Autodesk Inventor part; units mm, degrees
(part 2 of 2)
  arc A534 (36.3761, 13.3545) -> (36.8733, 13.0276) centre (36.8454, 13.5269) ccw
  arc A535 (36.3761, 13.3545) -> (36.3337, 13.4695) centre (0, 0) ccw
  arc A536 (36.4994, 14.041) -> (36.3337, 13.4695) centre (36.8025, 13.6433) ccw
  arc A537 (37.1579, 14.5094) -> (36.4994, 14.041) centre (43.9592, 4.2516) ccw
  arc A538 (37.1579, 14.5094) -> (37.2486, 14.5788) centre (36.7, 15.2016) ccw
  arc A539 (37.2486, 14.5788) -> (37.9831, 15.2771) centre (28.4355, 24.5841) ccw
  arc A540 (37.9831, 15.2771) -> (38.0042, 15.3845) centre (37.9115, 15.3469) ccw
  arc A541 (38.0042, 15.3845) -> (37.7515, 15.9946) centre (0, 0) ccw
  arc A542 (37.7515, 15.9946) -> (37.6607, 16.0555) centre (37.6594, 15.9556) ccw
  arc A543 (37.6607, 16.0555) -> (36.6475, 16.03) centre (37.4905, 2.7233) ccw
  arc A544 (36.6475, 16.03) -> (36.5343, 16.0149) centre (36.7, 15.2016) ccw
  arc A545 (35.7375, 15.8805) -> (36.5343, 16.0149) centre (34.0902, 28.0775) ccw
  arc A546 (35.2162, 16.1674) -> (35.7375, 15.8805) centre (35.6706, 16.376) ccw
  arc A547 (35.2162, 16.1674) -> (35.1649, 16.2787) centre (0, 0) ccw
  arc A548 (35.2853, 16.8614) -> (35.1649, 16.2787) centre (35.6186, 16.4887) ccw
  arc A549 (35.905, 17.38) -> (35.2853, 16.8614) centre (43.4901, 7.6875) ccw
  arc A550 (35.905, 17.38) -> (35.9899, 17.4564) centre (35.3942, 18.0342) ccw
  arc A551 (35.9899, 17.4564) -> (36.6674, 18.2102) centre (26.419, 26.7394) ccw
  arc A552 (36.6674, 18.2102) -> (36.68, 18.3188) centre (36.5905, 18.2741) ccw
  arc A553 (36.68, 18.3188) -> (36.3802, 18.9072) centre (0, 0) ccw
  arc A554 (36.3802, 18.9072) -> (36.2849, 18.9609) centre (36.2914, 18.8611) ccw
  arc A555 (36.2849, 18.9609) -> (35.2769, 18.8559) centre (37.1613, 5.6564) ccw
  arc A556 (35.2769, 18.8559) -> (35.1652, 18.832) centre (35.3942, 18.0342) ccw
  arc A557 (34.3813, 18.6355) -> (35.1652, 18.832) centre (31.7822, 30.6656) ccw
  arc A558 (33.8391, 18.8806) -> (34.3813, 18.6355) centre (34.2757, 19.1242) ccw
  arc A559 (33.8391, 18.8806) -> (33.7792, 18.9875) centre (0, 0) ccw
  arc A560 (33.8536, 19.5779) -> (33.7792, 18.9875) centre (34.2151, 19.2325) ccw
  arc A561 (34.4306, 20.1435) -> (33.8536, 19.5779) centre (42.7529, 11.076) ccw
  arc A562 (34.4306, 20.1435) -> (34.5094, 20.2263) centre (33.8701, 20.7556) ccw
  arc A563 (34.5094, 20.2263) -> (35.1256, 21.0309) centre (24.2396, 28.7298) ccw
  arc A564 (35.1256, 21.0309) -> (35.1296, 21.1402) centre (35.044, 21.0887) ccw
  arc A565 (35.1296, 21.1402) -> (34.7846, 21.7033) centre (0, 0) ccw
  arc A566 (34.7846, 21.7033) -> (34.6854, 21.7493) centre (34.6998, 21.6503) ccw
  arc A567 (34.6854, 21.7493) -> (33.6887, 21.5655) centre (36.6029, 8.5546) ccw
  arc A568 (33.6887, 21.5655) -> (33.5792, 21.533) centre (33.8701, 20.7556) ccw
  arc A569 (32.8132, 21.2756) -> (33.5792, 21.533) centre (29.2782, 33.0647) ccw
  arc A570 (32.2534, 21.4774) -> (32.8132, 21.2756) centre (32.6696, 21.7545) ccw
  arc A571 (32.2534, 21.4774) -> (32.1854, 21.5793) centre (0, 0) ccw
  arc A572 (32.2131, 22.1737) -> (32.1854, 21.5793) centre (32.6007, 21.8577) ccw
  arc A573 (32.7441, 22.7828) -> (32.2131, 22.1737) centre (41.7521, 14.3962) ccw
  arc A574 (32.7441, 22.7828) -> (32.8161, 22.8715) centre (32.1372, 23.3491) ccw
  arc A575 (32.8161, 22.8715) -> (33.3673, 23.722) centre (21.9107, 30.543) ccw
  arc A576 (33.3673, 23.722) -> (33.3627, 23.8313) centre (33.2813, 23.7732) ccw
  arc A577 (33.3627, 23.8313) -> (32.9745, 24.3655) centre (0, 0) ccw
  arc A578 (32.9745, 24.3655) -> (32.872, 24.4036) centre (32.8941, 24.3061) ccw
  arc A579 (32.872, 24.4036) -> (31.8928, 24.1422) centre (35.8189, 11.4) ccw
  arc A580 (31.8928, 24.1422) -> (31.7862, 24.1012) centre (32.1372, 23.3491) ccw
  arc A581 (31.0428, 23.7845) -> (31.7862, 24.1012) centre (26.5937, 35.2599) ccw
  arc A582 (30.4689, 23.9418) -> (31.0428, 23.7845) centre (30.8621, 24.2507) ccw
  arc A583 (30.4689, 23.9418) -> (30.3931, 24.038) centre (0, 0) ccw
  arc A584 (30.3741, 24.6327) -> (30.3931, 24.038) centre (30.7852, 24.3481) ccw
  arc A585 (30.8556, 25.2817) -> (30.3741, 24.6327) centre (40.4939, 17.6277) ccw
  arc A586 (30.8556, 25.2817) -> (30.9204, 25.3757) centre (30.2062, 25.7985) ccw
  arc A587 (30.9204, 25.3757) -> (31.4032, 26.2668) centre (19.4468, 32.168) ccw
  arc A588 (31.4032, 26.2668) -> (31.3901, 26.3754) centre (31.3135, 26.3111) ccw
  arc A589 (31.3901, 26.3754) -> (30.9612, 26.8776) centre (0, 0) ccw
  arc A590 (30.9612, 26.8776) -> (30.856, 26.9075) centre (30.8857, 26.812) ccw
  arc A591 (30.856, 26.9075) -> (29.9003, 26.5701) centre (34.8141, 14.1752) ccw
  arc A592 (29.9003, 26.5701) -> (29.7973, 26.5208) centre (30.2062, 25.7985) ccw
  arc A593 (29.081, 26.1468) -> (29.7973, 26.5208) centre (23.7453, 37.2377) ccw
  arc A594 (28.4965, 26.2585) -> (29.081, 26.1468) centre (28.8642, 26.5973) ccw
  arc A595 (28.4965, 26.2585) -> (28.4134, 26.3485) centre (0, 0) ccw
  arc A596 (28.3478, 26.9399) -> (28.4134, 26.3485) centre (28.78, 26.6885) ccw
  arc A597 (28.7769, 27.6246) -> (28.3478, 26.9399) centre (38.986, 20.7505) ccw
  arc A598 (28.7769, 27.6246) -> (28.8341, 27.7235) centre (28.089, 28.089) ccw
  arc A599 (28.8341, 27.7235) -> (29.2455, 28.6497) centre (16.863, 33.5946) ccw
  arc A600 (29.2455, 28.6497) -> (29.2239, 28.757) centre (29.1526, 28.6868) ccw
  arc A601 (29.2239, 28.757) -> (28.757, 29.2239) centre (0, 0) ccw
  arc A602 (28.757, 29.2239) -> (28.6497, 29.2455) centre (28.6868, 29.1526) ccw
  arc A603 (28.6497, 29.2455) -> (27.7235, 28.8341) centre (33.5946, 16.863) ccw
  arc A604 (27.7235, 28.8341) -> (27.6246, 28.7769) centre (28.089, 28.089) ccw
  arc A605 (26.9399, 28.3478) -> (27.6246, 28.7769) centre (20.7505, 38.986) ccw
  arc A606 (26.3485, 28.4134) -> (26.9399, 28.3478) centre (26.6885, 28.78) ccw
  arc A607 (26.3485, 28.4134) -> (26.2585, 28.4965) centre (0, 0) ccw
  arc A608 (26.1468, 29.081) -> (26.2585, 28.4965) centre (26.5973, 28.8642) ccw
  arc A609 (26.5208, 29.7973) -> (26.1468, 29.081) centre (37.2377, 23.7453) ccw
  arc A610 (26.5208, 29.7973) -> (26.5701, 29.9003) centre (25.7985, 30.2062) ccw
  arc A611 (26.5701, 29.9003) -> (26.9075, 30.856) centre (14.1752, 34.8141) ccw
  arc A612 (26.9075, 30.856) -> (26.8776, 30.9612) centre (26.812, 30.8857) ccw
  arc A613 (26.8776, 30.9612) -> (26.3754, 31.3901) centre (0, 0) ccw
  arc A614 (26.3754, 31.3901) -> (26.2668, 31.4032) centre (26.3111, 31.3135) ccw
  arc A615 (26.2668, 31.4032) -> (25.3757, 30.9204) centre (32.168, 19.4468) ccw
  arc A616 (25.3757, 30.9204) -> (25.2817, 30.8556) centre (25.7985, 30.2062) ccw
  arc A617 (24.6327, 30.3741) -> (25.2817, 30.8556) centre (17.6277, 40.4939) ccw
  arc A618 (24.038, 30.3931) -> (24.6327, 30.3741) centre (24.3481, 30.7852) ccw
  arc A619 (24.038, 30.3931) -> (23.9418, 30.4689) centre (0, 0) ccw
  arc A620 (23.7845, 31.0428) -> (23.9418, 30.4689) centre (24.2507, 30.8621) ccw
  arc A621 (24.1012, 31.7862) -> (23.7845, 31.0428) centre (35.2599, 26.5937) ccw
  arc A622 (24.1012, 31.7862) -> (24.1422, 31.8928) centre (23.3491, 32.1372) ccw
  arc A623 (24.1422, 31.8928) -> (24.4036, 32.872) centre (11.4, 35.8189) ccw
  arc A624 (24.4036, 32.872) -> (24.3655, 32.9745) centre (24.3061, 32.8941) ccw
  arc A625 (24.3655, 32.9745) -> (23.8313, 33.3627) centre (0, 0) ccw
  arc A626 (23.8313, 33.3627) -> (23.722, 33.3673) centre (23.7732, 33.2813) ccw
  arc A627 (23.722, 33.3673) -> (22.8715, 32.8161) centre (30.543, 21.9107) ccw
  arc A628 (22.8715, 32.8161) -> (22.7828, 32.7441) centre (23.3491, 32.1372) ccw
  arc A629 (22.1737, 32.2131) -> (22.7828, 32.7441) centre (14.3962, 41.7521) ccw
  arc A630 (21.5793, 32.1854) -> (22.1737, 32.2131) centre (21.8577, 32.6007) ccw
  arc A631 (21.5793, 32.1854) -> (21.4774, 32.2534) centre (0, 0) ccw
  arc A632 (21.2756, 32.8132) -> (21.4774, 32.2534) centre (21.7545, 32.6696) ccw
  arc A633 (21.533, 33.5792) -> (21.2756, 32.8132) centre (33.0647, 29.2782) ccw
  arc A634 (21.533, 33.5792) -> (21.5655, 33.6887) centre (20.7556, 33.8701) ccw
  arc A635 (21.5655, 33.6887) -> (21.7493, 34.6854) centre (8.5546, 36.6029) ccw
  arc A636 (21.7493, 34.6854) -> (21.7033, 34.7846) centre (21.6503, 34.6998) ccw
  arc A637 (21.7033, 34.7846) -> (21.1402, 35.1296) centre (0, 0) ccw
  arc A638 (21.1402, 35.1296) -> (21.0309, 35.1256) centre (21.0887, 35.044) ccw
  arc A639 (21.0309, 35.1256) -> (20.2263, 34.5094) centre (28.7298, 24.2396) ccw
  arc A640 (20.2263, 34.5094) -> (20.1435, 34.4306) centre (20.7556, 33.8701) ccw
  arc A641 (19.5779, 33.8536) -> (20.1435, 34.4306) centre (11.076, 42.7529) ccw
  arc A642 (18.9875, 33.7792) -> (19.5779, 33.8536) centre (19.2325, 34.2151) ccw
  arc A643 (18.9875, 33.7792) -> (18.8806, 33.8391) centre (0, 0) ccw
  arc A644 (18.6355, 34.3813) -> (18.8806, 33.8391) centre (19.1242, 34.2757) ccw
  arc A645 (18.832, 35.1652) -> (18.6355, 34.3813) centre (30.6656, 31.7822) ccw
  arc A646 (18.832, 35.1652) -> (18.8559, 35.2769) centre (18.0342, 35.3942) ccw
  arc A647 (18.8559, 35.2769) -> (18.9609, 36.2849) centre (5.6564, 37.1613) ccw
  arc A648 (18.9609, 36.2849) -> (18.9072, 36.3802) centre (18.8611, 36.2914) ccw
  arc A649 (18.9072, 36.3802) -> (18.3188, 36.68) centre (0, 0) ccw
  arc A650 (18.3188, 36.68) -> (18.2102, 36.6674) centre (18.2741, 36.5905) ccw
  arc A651 (18.2102, 36.6674) -> (17.4564, 35.9899) centre (26.7394, 26.419) ccw
  arc A652 (17.4564, 35.9899) -> (17.38, 35.905) centre (18.0342, 35.3942) ccw
  arc A653 (16.8614, 35.2853) -> (17.38, 35.905) centre (7.6875, 43.4901) ccw
  arc A654 (16.2787, 35.1649) -> (16.8614, 35.2853) centre (16.4887, 35.6186) ccw
  arc A655 (16.2787, 35.1649) -> (16.1674, 35.2162) centre (0, 0) ccw
  arc A656 (15.8805, 35.7375) -> (16.1674, 35.2162) centre (16.376, 35.6706) ccw
  arc A657 (16.0149, 36.5343) -> (15.8805, 35.7375) centre (28.0775, 34.0902) ccw
  arc A658 (16.0149, 36.5343) -> (16.03, 36.6475) centre (15.2016, 36.7) ccw
  arc A659 (16.03, 36.6475) -> (16.0555, 37.6607) centre (2.7233, 37.4905) ccw
  arc A660 (16.0555, 37.6607) -> (15.9946, 37.7515) centre (15.9556, 37.6594) ccw
  arc A661 (15.9946, 37.7515) -> (15.3845, 38.0042) centre (0, 0) ccw
  arc A662 (15.3845, 38.0042) -> (15.2771, 37.9831) centre (15.3469, 37.9115) ccw
  arc A663 (15.2771, 37.9831) -> (14.5788, 37.2486) centre (24.5841, 28.4355) ccw
  arc A664 (14.5788, 37.2486) -> (14.5094, 37.1579) centre (15.2016, 36.7) ccw
  arc A665 (14.041, 36.4994) -> (14.5094, 37.1579) centre (4.2516, 43.9592) ccw
  arc A666 (13.4695, 36.3337) -> (14.041, 36.4994) centre (13.6433, 36.8025) ccw
  arc A667 (13.4695, 36.3337) -> (13.3545, 36.3761) centre (0, 0) ccw
  arc A668 (13.0276, 36.8733) -> (13.3545, 36.3761) centre (13.5269, 36.8454) ccw
  arc A669 (13.0991, 37.6782) -> (13.0276, 36.8733) centre (25.3162, 36.1881) ccw
  arc A670 (13.0991, 37.6782) -> (13.1052, 37.7922) centre (12.2753, 37.7796) ccw
  arc A671 (13.1052, 37.7922) -> (13.0512, 38.8043) centre (-0.2266, 37.5886) ccw
  arc A672 (13.0512, 38.8043) -> (12.9833, 38.89) centre (12.9516, 38.7952) ccw
  arc A673 (12.9833, 38.89) -> (12.3553, 39.0941) centre (0, 0) ccw
  arc A674 (12.3553, 39.0941) -> (12.2499, 39.0646) centre (12.3251, 38.9987) ccw
  arc A675 (12.2499, 39.0646) -> (11.6114, 38.2776) centre (22.2773, 30.2767) ccw
  arc A676 (11.6114, 38.2776) -> (11.5493, 38.1817) centre (12.2753, 37.7796) ccw
  arc A677 (11.134, 37.4886) -> (11.5493, 38.1817) centre (0.7895, 44.1573) ccw
  arc A678 (10.5773, 37.2785) -> (11.134, 37.4886) centre (10.7137, 37.7595) ccw
  arc A679 (10.5773, 37.2785) -> (10.4593, 37.3117) centre (0, 0) ccw
  arc A680 (10.0944, 37.7817) -> (10.4593, 37.3117) centre (10.5943, 37.7932) ccw
  arc A681 (10.1025, 38.5898) -> (10.0944, 37.7817) centre (22.3989, 38.0628) ccw
  arc A682 (10.1025, 38.5898) -> (10.0997, 38.704) centre (9.2733, 38.6262) ccw
  arc A683 (10.0997, 38.704) -> (9.9664, 39.7087) centre (-3.175, 37.455) ccw
  arc A684 (9.9664, 39.7087) -> (9.892, 39.7888) centre (9.8679, 39.6917) ccw
  arc A685 (9.892, 39.7888) -> (9.2499, 39.943) centre (0, 0) ccw
  arc A686 (9.2499, 39.943) -> (9.1472, 39.9053) centre (9.2273, 39.8455) ccw
  arc A687 (9.1472, 39.9053) -> (8.5724, 39.0706) centre (19.8332, 31.9312) ccw
  arc A688 (8.5724, 39.0706) -> (8.518, 38.9702) centre (9.2733, 38.6262) ccw
  arc A689 (8.1583, 38.2466) -> (8.518, 38.9702) centre (-2.6774, 44.0831) ccw
  arc A690 (7.6198, 37.9934) -> (8.1583, 38.2466) centre (7.7181, 38.4837) ccw
  arc A691 (7.6198, 37.9934) -> (7.4997, 38.0173) centre (0, 0) ccw
  arc A692 (7.099, 38.4573) -> (7.4997, 38.0173) centre (7.5964, 38.5079) ccw
  arc A693 (7.0437, 39.2635) -> (7.099, 38.4573) centre (19.3435, 39.7029) ccw
  arc A694 (7.0437, 39.2635) -> (7.0319, 39.3771) centre (6.2142, 39.2347) ccw
  arc A695 (7.0319, 39.3771) -> (6.8202, 40.3682) centre (-6.1039, 37.0904) ccw
  arc A696 (6.8202, 40.3682) -> (6.7397, 40.4423) centre (6.7233, 40.3436) ccw
  arc A697 (6.7397, 40.4423) -> (6.0875, 40.5456) centre (0, 0) ccw
  arc A698 (6.0875, 40.5456) -> (5.988, 40.5) centre (6.0726, 40.4467) ccw
  arc A699 (5.988, 40.5) -> (5.4805, 39.6228) centre (17.2668, 33.3889) ccw
  arc A700 (5.4805, 39.6228) -> (5.4342, 39.5184) centre (6.2142, 39.2347) ccw
  arc A701 (5.1324, 38.7688) -> (5.4342, 39.5184) centre (-6.1279, 43.7371) ccw
  arc A702 (4.6154, 38.4742) -> (5.1324, 38.7688) centre (4.675, 38.9706) ccw
  arc A703 (4.6154, 38.4742) -> (4.4937, 38.4886) centre (0, 0) ccw
  arc A704 (4.0598, 38.8957) -> (4.4937, 38.4886) centre (4.5517, 38.9852) ccw
  arc A705 (3.9414, 39.6951) -> (4.0598, 38.8957) centre (16.1688, 41.0981) ccw
  arc A706 (3.9414, 39.6951) -> (3.9207, 39.8074) centre (3.1167, 39.6013) ccw
  arc A707 (3.9207, 39.8074) -> (3.6319, 40.7789) centre (-8.9952, 36.4972) ccw
  arc A708 (3.6319, 40.7789) -> (3.5459, 40.8464) centre (3.5372, 40.7468) ccw
  arc A709 (3.5459, 40.8464) -> (2.8876, 40.8982) centre (0, 0) ccw
  arc A710 (2.8876, 40.8982) -> (2.792, 40.845) centre (2.8805, 40.7984) ccw
  arc A711 (2.792, 40.845) -> (2.3548, 39.9306) centre (14.5939, 34.6407) ccw
  arc A712 (2.3548, 39.9306) -> (2.3168, 39.8229) centre (3.1167, 39.6013) ccw
  arc A713 (2.0748, 39.0519) -> (2.3168, 39.8229) centre (-9.5406, 43.1215) ccw
  arc A714 (1.5825, 38.7177) -> (2.0748, 39.0519) centre (1.6029, 39.2173) ccw
  arc A715 (1.5825, 38.7177) -> (1.4601, 38.7225) centre (0, 0) ccw
  arc A716 (0.9956, 39.0943) -> (1.4601, 38.7225) centre (1.4789, 39.2221) ccw
  arc A717 (0.8148, 39.8819) -> (0.9956, 39.0943) centre (12.8945, 42.24) ccw
  arc A718 (0.8148, 39.8819) -> (0.7853, 39.9923) centre (0, 39.7238) ccw
  arc A719 (0.7853, 39.9923) -> (0.4213, 40.9381) centre (-11.831, 35.6789) ccw
  arc A720 (0.4213, 40.9381) -> (0.3302, 40.9987) centre (0.3294, 40.8987) ccw
  arc A721 (0.3302, 40.9987) -> (-0.3302, 40.9987) centre (0, 0) ccw
  arc A722 (-0.3302, 40.9987) -> (-0.4213, 40.9381) centre (-0.3294, 40.8987) ccw
  arc A723 (-0.4213, 40.9381) -> (-0.7853, 39.9923) centre (11.831, 35.6789) ccw
  arc A724 (-0.7853, 39.9923) -> (-0.8148, 39.8819) centre (0, 39.7238) ccw
  arc A725 (-0.9956, 39.0943) -> (-0.8148, 39.8819) centre (-12.8945, 42.24) ccw
  arc A726 (-1.4601, 38.7225) -> (-0.9956, 39.0943) centre (-1.4789, 39.2221) ccw
  arc A727 (-1.4601, 38.7225) -> (-1.5825, 38.7177) centre (0, 0) ccw
  arc A728 (-2.0748, 39.0519) -> (-1.5825, 38.7177) centre (-1.6029, 39.2173) ccw
  arc A729 (-2.3168, 39.8229) -> (-2.0748, 39.0519) centre (9.5406, 43.1215) ccw
  arc A730 (-2.3168, 39.8229) -> (-2.3548, 39.9306) centre (-3.1167, 39.6013) ccw
  arc A731 (-2.3548, 39.9306) -> (-2.792, 40.845) centre (-14.5939, 34.6407) ccw
  arc A732 (-2.792, 40.845) -> (-2.8876, 40.8982) centre (-2.8805, 40.7984) ccw
  arc A733 (-2.8876, 40.8982) -> (-3.5459, 40.8464) centre (0, 0) ccw
  arc A734 (-3.5459, 40.8464) -> (-3.6319, 40.7789) centre (-3.5372, 40.7468) ccw
  arc A735 (-3.6319, 40.7789) -> (-3.9207, 39.8074) centre (8.9952, 36.4972) ccw
  arc A736 (-3.9207, 39.8074) -> (-3.9414, 39.6951) centre (-3.1167, 39.6013) ccw
  arc A737 (-4.0598, 38.8957) -> (-3.9414, 39.6951) centre (-16.1688, 41.0981) ccw
  arc A738 (-4.4937, 38.4886) -> (-4.0598, 38.8957) centre (-4.5517, 38.9852) ccw
  arc A739 (-4.4937, 38.4886) -> (-4.6154, 38.4742) centre (0, 0) ccw
  arc A740 (-5.1324, 38.7688) -> (-4.6154, 38.4742) centre (-4.675, 38.9706) ccw
  arc A741 (-5.4342, 39.5184) -> (-5.1324, 38.7688) centre (6.1279, 43.7371) ccw
  arc A742 (-5.4342, 39.5184) -> (-5.4805, 39.6228) centre (-6.2142, 39.2347) ccw
  arc A743 (-5.4805, 39.6228) -> (-5.988, 40.5) centre (-17.2668, 33.3889) ccw
  arc A744 (-5.988, 40.5) -> (-6.0875, 40.5456) centre (-6.0726, 40.4467) ccw
  arc A745 (-6.0875, 40.5456) -> (-6.7397, 40.4423) centre (0, 0) ccw
  arc A746 (-6.7397, 40.4423) -> (-6.8202, 40.3682) centre (-6.7233, 40.3436) ccw
  arc A747 (-6.8202, 40.3682) -> (-7.0319, 39.3771) centre (6.1039, 37.0904) ccw
  arc A748 (-7.0319, 39.3771) -> (-7.0437, 39.2635) centre (-6.2142, 39.2347) ccw
  arc A749 (-7.099, 38.4573) -> (-7.0437, 39.2635) centre (-19.3435, 39.7029) ccw
  arc A750 (-7.4997, 38.0173) -> (-7.099, 38.4573) centre (-7.5964, 38.5079) ccw
  arc A751 (-7.4997, 38.0173) -> (-7.6198, 37.9934) centre (0, 0) ccw
  arc A752 (-8.1583, 38.2466) -> (-7.6198, 37.9934) centre (-7.7181, 38.4837) ccw
  arc A753 (-8.518, 38.9702) -> (-8.1583, 38.2466) centre (2.6774, 44.0831) ccw
  arc A754 (-8.518, 38.9702) -> (-8.5724, 39.0706) centre (-9.2733, 38.6262) ccw
  arc A755 (-8.5724, 39.0706) -> (-9.1472, 39.9053) centre (-19.8332, 31.9312) ccw
  arc A756 (-9.1472, 39.9053) -> (-9.2499, 39.943) centre (-9.2273, 39.8455) ccw
  arc A757 (-9.2499, 39.943) -> (-9.892, 39.7888) centre (0, 0) ccw
  arc A758 (-9.892, 39.7888) -> (-9.9664, 39.7087) centre (-9.8679, 39.6917) ccw
  arc A759 (-9.9664, 39.7087) -> (-10.0997, 38.704) centre (3.175, 37.455) ccw
  arc A760 (-10.0997, 38.704) -> (-10.1025, 38.5898) centre (-9.2733, 38.6262) ccw
  arc A761 (-10.0944, 37.7817) -> (-10.1025, 38.5898) centre (-22.3989, 38.0628) ccw
  arc A762 (-10.4593, 37.3117) -> (-10.0944, 37.7817) centre (-10.5943, 37.7932) ccw
  arc A763 (-10.4593, 37.3117) -> (-10.5773, 37.2785) centre (0, 0) ccw
  arc A764 (-11.134, 37.4886) -> (-10.5773, 37.2785) centre (-10.7137, 37.7595) ccw
  arc A765 (-11.5493, 38.1817) -> (-11.134, 37.4886) centre (-0.7895, 44.1573) ccw
  arc A766 (-11.5493, 38.1817) -> (-11.6114, 38.2776) centre (-12.2753, 37.7796) ccw
  arc A767 (-11.6114, 38.2776) -> (-12.2499, 39.0646) centre (-22.2773, 30.2767) ccw
  arc A768 (-12.2499, 39.0646) -> (-12.3553, 39.0941) centre (-12.3251, 38.9987) ccw
  arc A769 (-12.3553, 39.0941) -> (-12.9833, 38.89) centre (0, 0) ccw
  arc A770 (-12.9833, 38.89) -> (-13.0512, 38.8043) centre (-12.9516, 38.7952) ccw
  arc A771 (-13.0512, 38.8043) -> (-13.1052, 37.7922) centre (0.2266, 37.5886) ccw
  arc A772 (-13.1052, 37.7922) -> (-13.0991, 37.6782) centre (-12.2753, 37.7796) ccw
  arc A773 (-13.0276, 36.8733) -> (-13.0991, 37.6782) centre (-25.3162, 36.1881) ccw
  arc A774 (-13.3545, 36.3761) -> (-13.0276, 36.8733) centre (-13.5269, 36.8454) ccw
  arc A775 (-13.3545, 36.3761) -> (-13.4695, 36.3337) centre (0, 0) ccw
  arc A776 (-14.041, 36.4994) -> (-13.4695, 36.3337) centre (-13.6433, 36.8025) ccw
  arc A777 (-14.5094, 37.1579) -> (-14.041, 36.4994) centre (-4.2516, 43.9592) ccw
  arc A778 (-14.5094, 37.1579) -> (-14.5788, 37.2486) centre (-15.2016, 36.7) ccw
  arc A779 (-14.5788, 37.2486) -> (-15.2771, 37.9831) centre (-24.5841, 28.4355) ccw
  arc A780 (-15.2771, 37.9831) -> (-15.3845, 38.0042) centre (-15.3469, 37.9115) ccw
  arc A781 (-15.3845, 38.0042) -> (-15.9946, 37.7515) centre (0, 0) ccw
  arc A782 (-15.9946, 37.7515) -> (-16.0555, 37.6607) centre (-15.9556, 37.6594) ccw
  arc A783 (-16.0555, 37.6607) -> (-16.03, 36.6475) centre (-2.7233, 37.4905) ccw
  arc A784 (-16.03, 36.6475) -> (-16.0149, 36.5343) centre (-15.2016, 36.7) ccw
  arc A785 (-15.8805, 35.7375) -> (-16.0149, 36.5343) centre (-28.0775, 34.0902) ccw
  arc A786 (-16.1674, 35.2162) -> (-15.8805, 35.7375) centre (-16.376, 35.6706) ccw
  arc A787 (-16.1674, 35.2162) -> (-16.2787, 35.1649) centre (0, 0) ccw
  arc A788 (-16.8614, 35.2853) -> (-16.2787, 35.1649) centre (-16.4887, 35.6186) ccw
  arc A789 (-17.38, 35.905) -> (-16.8614, 35.2853) centre (-7.6875, 43.4901) ccw
  arc A790 (-17.38, 35.905) -> (-17.4564, 35.9899) centre (-18.0342, 35.3942) ccw
  arc A791 (-17.4564, 35.9899) -> (-18.2102, 36.6674) centre (-26.7394, 26.419) ccw
  arc A792 (-18.2102, 36.6674) -> (-18.3188, 36.68) centre (-18.2741, 36.5905) ccw
  arc A793 (-18.3188, 36.68) -> (-18.9072, 36.3802) centre (0, 0) ccw
  arc A794 (-18.9072, 36.3802) -> (-18.9609, 36.2849) centre (-18.8611, 36.2914) ccw
  arc A795 (-18.9609, 36.2849) -> (-18.8559, 35.2769) centre (-5.6564, 37.1613) ccw
  arc A796 (-18.8559, 35.2769) -> (-18.832, 35.1652) centre (-18.0342, 35.3942) ccw
  arc A797 (-18.6355, 34.3813) -> (-18.832, 35.1652) centre (-30.6656, 31.7822) ccw
  arc A798 (-18.8806, 33.8391) -> (-18.6355, 34.3813) centre (-19.1242, 34.2757) ccw
  arc A799 (-18.8806, 33.8391) -> (-18.9875, 33.7792) centre (0, 0) ccw
  arc A800 (-19.5779, 33.8536) -> (-18.9875, 33.7792) centre (-19.2325, 34.2151) ccw
  arc A801 (-20.1435, 34.4306) -> (-19.5779, 33.8536) centre (-11.076, 42.7529) ccw
  arc A802 (-20.1435, 34.4306) -> (-20.2263, 34.5094) centre (-20.7556, 33.8701) ccw
  arc A803 (-20.2263, 34.5094) -> (-21.0309, 35.1256) centre (-28.7298, 24.2396) ccw
  arc A804 (-21.0309, 35.1256) -> (-21.1402, 35.1296) centre (-21.0887, 35.044) ccw
  arc A805 (-21.1402, 35.1296) -> (-21.7033, 34.7846) centre (0, 0) ccw
  arc A806 (-21.7033, 34.7846) -> (-21.7493, 34.6854) centre (-21.6503, 34.6998) ccw
  arc A807 (-21.7493, 34.6854) -> (-21.5655, 33.6887) centre (-8.5546, 36.6029) ccw
  arc A808 (-21.5655, 33.6887) -> (-21.533, 33.5792) centre (-20.7556, 33.8701) ccw
  arc A809 (-21.2756, 32.8132) -> (-21.533, 33.5792) centre (-33.0647, 29.2782) ccw
  arc A810 (-21.4774, 32.2534) -> (-21.2756, 32.8132) centre (-21.7545, 32.6696) ccw
  arc A811 (-21.4774, 32.2534) -> (-21.5793, 32.1854) centre (0, 0) ccw
  arc A812 (-22.1737, 32.2131) -> (-21.5793, 32.1854) centre (-21.8577, 32.6007) ccw
  arc A813 (-22.7828, 32.7441) -> (-22.1737, 32.2131) centre (-14.3962, 41.7521) ccw
  arc A814 (-22.7828, 32.7441) -> (-22.8715, 32.8161) centre (-23.3491, 32.1372) ccw
  arc A815 (-22.8715, 32.8161) -> (-23.722, 33.3673) centre (-30.543, 21.9107) ccw
  arc A816 (-23.722, 33.3673) -> (-23.8313, 33.3627) centre (-23.7732, 33.2813) ccw
  arc A817 (-23.8313, 33.3627) -> (-24.3655, 32.9745) centre (0, 0) ccw
  arc A818 (-24.3655, 32.9745) -> (-24.4036, 32.872) centre (-24.3061, 32.8941) ccw
  arc A819 (-24.4036, 32.872) -> (-24.1422, 31.8928) centre (-11.4, 35.8189) ccw
  arc A820 (-24.1422, 31.8928) -> (-24.1012, 31.7862) centre (-23.3491, 32.1372) ccw
  arc A821 (-23.7845, 31.0428) -> (-24.1012, 31.7862) centre (-35.2599, 26.5937) ccw
  arc A822 (-23.9418, 30.4689) -> (-23.7845, 31.0428) centre (-24.2507, 30.8621) ccw
  arc A823 (-23.9418, 30.4689) -> (-24.038, 30.3931) centre (0, 0) ccw
  arc A824 (-24.6327, 30.3741) -> (-24.038, 30.3931) centre (-24.3481, 30.7852) ccw
  arc A825 (-25.2817, 30.8556) -> (-24.6327, 30.3741) centre (-17.6277, 40.4939) ccw
  arc A826 (-25.2817, 30.8556) -> (-25.3757, 30.9204) centre (-25.7985, 30.2062) ccw
  arc A827 (-25.3757, 30.9204) -> (-26.2668, 31.4032) centre (-32.168, 19.4468) ccw
  arc A828 (-26.2668, 31.4032) -> (-26.3754, 31.3901) centre (-26.3111, 31.3135) ccw
  arc A829 (-26.3754, 31.3901) -> (-26.8776, 30.9612) centre (0, 0) ccw
  arc A830 (-26.8776, 30.9612) -> (-26.9075, 30.856) centre (-26.812, 30.8857) ccw
  arc A831 (-26.9075, 30.856) -> (-26.5701, 29.9003) centre (-14.1752, 34.8141) ccw
  arc A832 (-26.5701, 29.9003) -> (-26.5208, 29.7973) centre (-25.7985, 30.2062) ccw
  arc A833 (-26.1468, 29.081) -> (-26.5208, 29.7973) centre (-37.2377, 23.7453) ccw
  arc A834 (-26.2585, 28.4965) -> (-26.1468, 29.081) centre (-26.5973, 28.8642) ccw
  arc A835 (-26.2585, 28.4965) -> (-26.3485, 28.4134) centre (0, 0) ccw
  arc A836 (-26.9399, 28.3478) -> (-26.3485, 28.4134) centre (-26.6885, 28.78) ccw
  arc A837 (-27.6246, 28.7769) -> (-26.9399, 28.3478) centre (-20.7505, 38.986) ccw
  arc A838 (-27.6246, 28.7769) -> (-27.7235, 28.8341) centre (-28.089, 28.089) ccw
  arc A839 (-27.7235, 28.8341) -> (-28.6497, 29.2455) centre (-33.5946, 16.863) ccw
  arc A840 (-28.6497, 29.2455) -> (-28.757, 29.2239) centre (-28.6868, 29.1526) ccw
  arc A841 (-28.757, 29.2239) -> (-29.2239, 28.757) centre (0, 0) ccw
  arc A842 (-29.2239, 28.757) -> (-29.2455, 28.6497) centre (-29.1526, 28.6868) ccw
  arc A843 (-29.2455, 28.6497) -> (-28.8341, 27.7235) centre (-16.863, 33.5946) ccw
  arc A844 (-28.8341, 27.7235) -> (-28.7769, 27.6246) centre (-28.089, 28.089) ccw
  arc A845 (-28.3478, 26.9399) -> (-28.7769, 27.6246) centre (-38.986, 20.7505) ccw
  arc A846 (-28.4134, 26.3485) -> (-28.3478, 26.9399) centre (-28.78, 26.6885) ccw
  arc A847 (-28.4134, 26.3485) -> (-28.4965, 26.2585) centre (0, 0) ccw
  arc A848 (-29.081, 26.1468) -> (-28.4965, 26.2585) centre (-28.8642, 26.5973) ccw
  arc A849 (-29.7973, 26.5208) -> (-29.081, 26.1468) centre (-23.7453, 37.2377) ccw
  arc A850 (-29.7973, 26.5208) -> (-29.9003, 26.5701) centre (-30.2062, 25.7985) ccw
  arc A851 (-29.9003, 26.5701) -> (-30.856, 26.9075) centre (-34.8141, 14.1752) ccw
  arc A852 (-30.856, 26.9075) -> (-30.9612, 26.8776) centre (-30.8857, 26.812) ccw
  arc A853 (-30.9612, 26.8776) -> (-31.3901, 26.3754) centre (0, 0) ccw
  arc A854 (-31.3901, 26.3754) -> (-31.4032, 26.2668) centre (-31.3135, 26.3111) ccw
  arc A855 (-31.4032, 26.2668) -> (-30.9204, 25.3757) centre (-19.4468, 32.168) ccw
  arc A856 (-30.9204, 25.3757) -> (-30.8556, 25.2817) centre (-30.2062, 25.7985) ccw
  arc A857 (-30.3741, 24.6327) -> (-30.8556, 25.2817) centre (-40.4939, 17.6277) ccw
  arc A858 (-30.3931, 24.038) -> (-30.3741, 24.6327) centre (-30.7852, 24.3481) ccw
  arc A859 (-30.3931, 24.038) -> (-30.4689, 23.9418) centre (0, 0) ccw
  arc A860 (-31.0428, 23.7845) -> (-30.4689, 23.9418) centre (-30.8621, 24.2507) ccw
  arc A861 (-31.7862, 24.1012) -> (-31.0428, 23.7845) centre (-26.5937, 35.2599) ccw
  arc A862 (-31.7862, 24.1012) -> (-31.8928, 24.1422) centre (-32.1372, 23.3491) ccw
  arc A863 (-31.8928, 24.1422) -> (-32.872, 24.4036) centre (-35.8189, 11.4) ccw
  arc A864 (-32.872, 24.4036) -> (-32.9745, 24.3655) centre (-32.8941, 24.3061) ccw
  arc A865 (-32.9745, 24.3655) -> (-33.3627, 23.8313) centre (0, 0) ccw
  arc A866 (-33.3627, 23.8313) -> (-33.3673, 23.722) centre (-33.2813, 23.7732) ccw
  arc A867 (-33.3673, 23.722) -> (-32.8161, 22.8715) centre (-21.9107, 30.543) ccw
  arc A868 (-32.8161, 22.8715) -> (-32.7441, 22.7828) centre (-32.1372, 23.3491) ccw
  arc A869 (-32.2131, 22.1737) -> (-32.7441, 22.7828) centre (-41.7521, 14.3962) ccw
  arc A870 (-32.1854, 21.5793) -> (-32.2131, 22.1737) centre (-32.6007, 21.8577) ccw
  arc A871 (-32.1854, 21.5793) -> (-32.2534, 21.4774) centre (0, 0) ccw
  arc A872 (-32.8132, 21.2756) -> (-32.2534, 21.4774) centre (-32.6696, 21.7545) ccw
  arc A873 (-33.5792, 21.533) -> (-32.8132, 21.2756) centre (-29.2782, 33.0647) ccw
  arc A874 (-33.5792, 21.533) -> (-33.6887, 21.5655) centre (-33.8701, 20.7556) ccw
  arc A875 (-33.6887, 21.5655) -> (-34.6854, 21.7493) centre (-36.6029, 8.5546) ccw
  arc A876 (-34.6854, 21.7493) -> (-34.7846, 21.7033) centre (-34.6998, 21.6503) ccw
  arc A877 (-34.7846, 21.7033) -> (-35.1296, 21.1402) centre (0, 0) ccw
  arc A878 (-35.1296, 21.1402) -> (-35.1256, 21.0309) centre (-35.044, 21.0887) ccw
  arc A879 (-35.1256, 21.0309) -> (-34.5094, 20.2263) centre (-24.2396, 28.7298) ccw
  arc A880 (-34.5094, 20.2263) -> (-34.4306, 20.1435) centre (-33.8701, 20.7556) ccw
  arc A881 (-33.8536, 19.5779) -> (-34.4306, 20.1435) centre (-42.7529, 11.076) ccw
  arc A882 (-33.7792, 18.9875) -> (-33.8536, 19.5779) centre (-34.2151, 19.2325) ccw
  arc A883 (-33.7792, 18.9875) -> (-33.8391, 18.8806) centre (0, 0) ccw
  arc A884 (-34.3813, 18.6355) -> (-33.8391, 18.8806) centre (-34.2757, 19.1242) ccw
  arc A885 (-35.1652, 18.832) -> (-34.3813, 18.6355) centre (-31.7822, 30.6656) ccw
  arc A886 (-35.1652, 18.832) -> (-35.2769, 18.8559) centre (-35.3942, 18.0342) ccw
  arc A887 (-35.2769, 18.8559) -> (-36.2849, 18.9609) centre (-37.1613, 5.6564) ccw
  arc A888 (-36.2849, 18.9609) -> (-36.3802, 18.9072) centre (-36.2914, 18.8611) ccw
  arc A889 (-36.3802, 18.9072) -> (-36.68, 18.3188) centre (0, 0) ccw
  arc A890 (-36.68, 18.3188) -> (-36.6674, 18.2102) centre (-36.5905, 18.2741) ccw
  arc A891 (-36.6674, 18.2102) -> (-35.9899, 17.4564) centre (-26.419, 26.7394) ccw
  arc A892 (-35.9899, 17.4564) -> (-35.905, 17.38) centre (-35.3942, 18.0342) ccw
  arc A893 (-35.2853, 16.8614) -> (-35.905, 17.38) centre (-43.4901, 7.6875) ccw
  arc A894 (-35.1649, 16.2787) -> (-35.2853, 16.8614) centre (-35.6186, 16.4887) ccw
  arc A895 (-35.1649, 16.2787) -> (-35.2162, 16.1674) centre (0, 0) ccw
  arc A896 (-35.7375, 15.8805) -> (-35.2162, 16.1674) centre (-35.6706, 16.376) ccw
  arc A897 (-36.5343, 16.0149) -> (-35.7375, 15.8805) centre (-34.0902, 28.0775) ccw
  arc A898 (-36.5343, 16.0149) -> (-36.6475, 16.03) centre (-36.7, 15.2016) ccw
  arc A899 (-36.6475, 16.03) -> (-37.6607, 16.0555) centre (-37.4905, 2.7233) ccw
  arc A900 (-37.6607, 16.0555) -> (-37.7515, 15.9946) centre (-37.6594, 15.9556) ccw
  arc A901 (-37.7515, 15.9946) -> (-38.0042, 15.3845) centre (0, 0) ccw
  arc A902 (-38.0042, 15.3845) -> (-37.9831, 15.2771) centre (-37.9115, 15.3469) ccw
  arc A903 (-37.9831, 15.2771) -> (-37.2486, 14.5788) centre (-28.4355, 24.5841) ccw
  arc A904 (-37.2486, 14.5788) -> (-37.1579, 14.5094) centre (-36.7, 15.2016) ccw
  arc A905 (-36.4994, 14.041) -> (-37.1579, 14.5094) centre (-43.9592, 4.2516) ccw
  arc A906 (-36.3337, 13.4695) -> (-36.4994, 14.041) centre (-36.8025, 13.6433) ccw
  arc A907 (-36.3337, 13.4695) -> (-36.3761, 13.3545) centre (0, 0) ccw
  arc A908 (-36.8733, 13.0276) -> (-36.3761, 13.3545) centre (-36.8454, 13.5269) ccw
  arc A909 (-37.6782, 13.0991) -> (-36.8733, 13.0276) centre (-36.1881, 25.3162) ccw
  arc A910 (-37.6782, 13.0991) -> (-37.7922, 13.1052) centre (-37.7796, 12.2753) ccw
  arc A911 (-37.7922, 13.1052) -> (-38.8043, 13.0512) centre (-37.5886, -0.2266) ccw
  arc A912 (-38.8043, 13.0512) -> (-38.89, 12.9833) centre (-38.7952, 12.9516) ccw
  arc A913 (-38.89, 12.9833) -> (-39.0941, 12.3553) centre (0, 0) ccw
  arc A914 (-39.0941, 12.3553) -> (-39.0646, 12.2499) centre (-38.9987, 12.3251) ccw
  arc A915 (-39.0646, 12.2499) -> (-38.2776, 11.6114) centre (-30.2767, 22.2773) ccw
  arc A916 (-38.2776, 11.6114) -> (-38.1817, 11.5493) centre (-37.7796, 12.2753) ccw
  arc A917 (-37.4886, 11.134) -> (-38.1817, 11.5493) centre (-44.1573, 0.7895) ccw
  arc A918 (-37.2785, 10.5773) -> (-37.4886, 11.134) centre (-37.7595, 10.7137) ccw
  arc A919 (-37.2785, 10.5773) -> (-37.3117, 10.4593) centre (0, 0) ccw
  arc A920 (-37.7817, 10.0944) -> (-37.3117, 10.4593) centre (-37.7932, 10.5943) ccw
  arc A921 (-38.5898, 10.1025) -> (-37.7817, 10.0944) centre (-38.0628, 22.3989) ccw
  arc A922 (-38.5898, 10.1025) -> (-38.704, 10.0997) centre (-38.6262, 9.2733) ccw
  arc A923 (-38.704, 10.0997) -> (-39.7087, 9.9664) centre (-37.455, -3.175) ccw
  arc A924 (-39.7087, 9.9664) -> (-39.7888, 9.892) centre (-39.6917, 9.8679) ccw
  arc A925 (-39.7888, 9.892) -> (-39.943, 9.2499) centre (0, 0) ccw
  arc A926 (-39.943, 9.2499) -> (-39.9053, 9.1472) centre (-39.8455, 9.2273) ccw
  arc A927 (-39.9053, 9.1472) -> (-39.0706, 8.5724) centre (-31.9312, 19.8332) ccw
  arc A928 (-39.0706, 8.5724) -> (-38.9702, 8.518) centre (-38.6262, 9.2733) ccw
  arc A929 (-38.2466, 8.1583) -> (-38.9702, 8.518) centre (-44.0831, -2.6774) ccw
  arc A930 (-37.9934, 7.6198) -> (-38.2466, 8.1583) centre (-38.4837, 7.7181) ccw
  arc A931 (-37.9934, 7.6198) -> (-38.0173, 7.4997) centre (0, 0) ccw
  arc A932 (-38.4573, 7.099) -> (-38.0173, 7.4997) centre (-38.5079, 7.5964) ccw
  arc A933 (-39.2635, 7.0437) -> (-38.4573, 7.099) centre (-39.7029, 19.3435) ccw
  arc A934 (-39.2635, 7.0437) -> (-39.3771, 7.0319) centre (-39.2347, 6.2142) ccw
  arc A935 (-39.3771, 7.0319) -> (-40.3682, 6.8202) centre (-37.0904, -6.1039) ccw
  arc A936 (-40.3682, 6.8202) -> (-40.4423, 6.7397) centre (-40.3436, 6.7233) ccw
  arc A937 (-40.4423, 6.7397) -> (-40.5456, 6.0875) centre (0, 0) ccw
  arc A938 (-40.5456, 6.0875) -> (-40.5, 5.988) centre (-40.4467, 6.0726) ccw
  arc A939 (-40.5, 5.988) -> (-39.6228, 5.4805) centre (-33.3889, 17.2668) ccw
  arc A940 (-39.6228, 5.4805) -> (-39.5184, 5.4342) centre (-39.2347, 6.2142) ccw
  arc A941 (-38.7688, 5.1324) -> (-39.5184, 5.4342) centre (-43.7371, -6.1279) ccw
  arc A942 (-38.4742, 4.6154) -> (-38.7688, 5.1324) centre (-38.9706, 4.675) ccw
  arc A943 (-38.4742, 4.6154) -> (-38.4886, 4.4937) centre (0, 0) ccw
  arc A944 (-38.8957, 4.0598) -> (-38.4886, 4.4937) centre (-38.9852, 4.5517) ccw
  arc A945 (-39.6951, 3.9414) -> (-38.8957, 4.0598) centre (-41.0981, 16.1688) ccw
  arc A946 (-39.6951, 3.9414) -> (-39.8074, 3.9207) centre (-39.6013, 3.1167) ccw
  arc A947 (-39.8074, 3.9207) -> (-40.7789, 3.6319) centre (-36.4972, -8.9952) ccw
  arc A948 (-40.7789, 3.6319) -> (-40.8464, 3.5459) centre (-40.7468, 3.5372) ccw
  arc A949 (-40.8464, 3.5459) -> (-40.8982, 2.8875) centre (0, 0) ccw
  arc A950 (-40.8982, 2.8875) -> (-40.845, 2.792) centre (-40.7984, 2.8805) ccw
  arc A951 (-40.845, 2.792) -> (-39.9306, 2.3548) centre (-34.6407, 14.5939) ccw
  arc A952 (-39.9306, 2.3548) -> (-39.8229, 2.3168) centre (-39.6013, 3.1167) ccw
  arc A953 (-39.0519, 2.0748) -> (-39.8229, 2.3168) centre (-43.1215, -9.5406) ccw
  arc A954 (-38.7177, 1.5825) -> (-39.0519, 2.0748) centre (-39.2173, 1.6029) ccw
  arc A955 (-38.7177, 1.5825) -> (-38.7225, 1.4601) centre (0, 0) ccw
  arc A956 (-39.0943, 0.9956) -> (-38.7225, 1.4601) centre (-39.2221, 1.4789) ccw
  arc A957 (-39.8819, 0.8148) -> (-39.0943, 0.9956) centre (-42.24, 12.8945) ccw
  arc A958 (-39.8819, 0.8148) -> (-39.9923, 0.7853) centre (-39.7238, 0) ccw
  arc A959 (-39.9923, 0.7853) -> (-40.9381, 0.4213) centre (-35.6789, -11.831) ccw
  arc A960 (-40.9381, 0.4213) -> (-40.9987, 0.3302) centre (-40.8987, 0.3294) ccw
  constraints: 1920 point on circle, 961 centre point
extrude "Extrusion1" cut sketch "_____12" against normal blind 10
sketch "Sketch3" plane through (0, 0, -10) normal (0, 0, -1) x (-0.9969, 0.0785, 0)
  point P0 (0, 0)
hole "Hole1" at (0, 0, -10) direction (0, 0, 1) diameter 20 depth 10
sketch "_____5" plane through (0, 0, 0) normal (1, 0, 0) x (0, 0, -1)
  line L0 (500, 0) -> (-500, 0)
  line L1 (9.7, 10) -> (10, 10)
  line L2 (10, 10) -> (10, 10.3)
  line L3 (10, 10.3) -> (9.7, 10)
  constraints: 8 end point
revolve "Revolution2" cut sketch "_____5" angle 360 about axis through (0, 0, -500) along (0, 0, -1)
sketch "_____13" plane through (0, 0, 0) normal (1, 0, 0) x (0, 0, -1)
  line L0 (500, 0) -> (-500, 0)
  line L1 (0, 10.3) -> (0, 10)
  line L2 (0, 10) -> (0.3, 10)
  line L3 (0.3, 10) -> (0, 10.3)
  constraints: 8 end point
revolve "Revolution3" cut sketch "_____13" angle 360 about axis through (0, 0, -500) along (0, 0, -1)
sketch "Sketch6" plane through (0, 0, -10) normal (0, 0, -1) x (-0.9969, 0.0785, 0)
  point P0 (-9.7417, 11.4061)
hole "Hole2" at (10.6066, 10.6066, -10) direction (0, 0, 1) diameter 3 depth 10
pattern_linear "Rectangular Pattern1" count 2 spacing 21.2132 along (-1, 0, 0) count 2 spacing 21.2132 along (0, -1, 0) of "Hole2"
body "Solid1"
